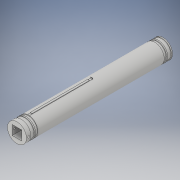
# Autodesk Inventor part: Axel_SBail
Saved by Autodesk Inventor 2019 (Build 230136000, 136)
## iProperties
Created: 2019-04-10
Part Number: Axel_SBail
Material: Generic
Document SubType Name: Modeling
Designer: samson.bailor
Density: 1 g/cm^3
Appearance: Default
Author: samson.bailor
Autodesk Inventor part; units mm, degrees
ref_plane "YZ Plane" through (0, 0, 0) normal (1, 0, 0) x (0, 1, 0)
ref_plane "XZ Plane" through (0, 0, 0) normal (0, 1, 0) x (-1, 0, 0)
ref_plane "XY Plane" through (0, 0, 0) normal (0, 0, 1) x (1, 0, 0)
sketch "Sketch1" plane through (0, 0, 0) normal (0, 0, 1) x (1, 0, 0)
  circle A0 centre (0, 0) radius 25.4
  dimension "d0" = 50.8
  constraints: 1 centre point, 1 coincident
  measures "d0" diameter of A0
extrude "Extrusion1" add sketch "Sketch1" along normal blind 355.6
sketch "Sketch4" plane through (0, 0, 355.6) normal (0, 0, 1) x (1, 0, 0)
  line L0 (31.0854, 16.4706) -> (47.788, 16.4706)
  line L1 (47.788, 16.4706) -> (47.788, 0)
  line L2 (47.788, 0) -> (31.0854, 0)
  line L3 (31.0854, 0) -> (31.0854, 16.4706)
  point P0 (0, 0)
  constraints: 8 end point, 2 parallel, 1 horizontal, 1 perpendicular
extrude "Extrusion4" add sketch "Sketch4" against normal blind 3.175
sketch "Sketch5" plane through (0, 0, 352.425) normal (0, 0, -1) x (-1, 0, 0)
  circle A0 centre (0, 0) radius 25.4
  circle A1 centre (0, 0) radius 23.8125
  dimension "d19" = 1.5875
  constraints: 2 centre point, 1 coincident
  measures "d19" radial gap between concentric circles of A0 A1
extrude "Extrusion5" cut sketch "Sketch5" along normal blind 6.35
sketch "Sketch6" plane through (0, 0, 0) normal (0, 0, -1) x (-1, 0, 0)
  line L0 (29.0417, -43.641) -> (10.5178, -43.641)
  line L1 (10.5178, -43.641) -> (10.5178, -69.3861)
  line L2 (10.5178, -69.3861) -> (29.0417, -69.3861)
  line L3 (29.0417, -69.3861) -> (29.0417, -43.641)
  point P0 (0, 0)
  constraints: 8 end point, 2 parallel, 1 horizontal, 1 perpendicular
extrude "Extrusion6" add sketch "Sketch6" against normal blind 3.175
sketch "Sketch7" plane through (0, 0, 3.175) normal (0, 0, 1) x (1, 0, 0)
  circle A0 centre (0, 0) radius 25.4
  circle A1 centre (0, 0) radius 23.8125
  constraints: 2 centre point, 2 coincident
extrude "Extrusion7" cut sketch "Sketch7" along normal blind 6.35
sketch "Sketch8" plane through (-29.0417, -69.3861, 0) normal (-1, 0, 0) x (0, 0, 1)
  line L0 (0, 0) -> (0, 25.7451) projected
  line L1 (3.175, 25.7451) -> (3.175, 0) projected
  line L2 (0, 0) -> (3.175, 0)
  line L3 (3.175, 0) -> (3.175, 25.7451)
  line L4 (3.175, 25.7451) -> (0, 25.7451)
  line L5 (0, 25.7451) -> (0, 0)
  point P0 (0, 69.3861)
  constraints: 8 end point, 2 parallel, 1 horizontal, 1 perpendicular
extrude "Extrusion8" cut sketch "Sketch8" against normal through all
sketch "Sketch9" plane through (0, 0, 355.6) normal (0, 0, 1) x (1, 0, 0)
  line L0 (31.0854, 16.4706) -> (47.788, 16.4706) projected
  line L1 (31.0854, 16.4706) -> (47.788, 16.4706)
  line L2 (47.788, 16.4706) -> (47.788, 0)
  line L3 (47.788, 0) -> (31.0854, 0)
  line L4 (31.0854, 0) -> (31.0854, 16.4706)
  point P0 (0, 0)
  constraints: 8 end point, 2 parallel, 1 horizontal, 1 perpendicular
extrude "Extrusion9" cut sketch "Sketch9" against normal blind 6.35
sketch "Sketch10" plane through (0, 0, 346.075) normal (0, 0, 1) x (1, 0, 0)
  circle A0 centre (0, 0) radius 25.4 projected
  line L0 (2.54, 25.4) -> (2.54, 26.67)
  line L1 (2.54, 26.67) -> (0, 26.67)
  line L2 (0, 26.67) -> (0, 25.4)
  line L3 (-2.54, 25.4) -> (-2.54, 26.67)
  line L4 (-2.54, 26.67) -> (0, 26.67)
  line L5 (0, 26.67) -> (0, 25.4)
  arc A1 (2.54, 25.2727) -> (-2.54, 25.2727) centre (0, 0) ccw
  line L6 (2.54, 25.4) -> (2.54, 25.2727)
  line L7 (-2.54, 25.4) -> (-2.54, 25.2727)
  dimension "d30" = 2.54
  dimension "d31" = 1.27
  dimension "d32" = 2.54
  dimension "d33" = 1.27
  constraints: 16 end point, 3 point on circle, 2 parallel, 2 vertical, 1 centre point, 1 vertical alignment, 1 other
  measures "d30" distance of L1.end L0.end
  measures "d31" distance of L0.end L0.start
  measures "d32" distance of L3.end L4.end
  measures "d33" distance of L3.start L3.end
extrude "Extrusion10" add sketch "Sketch10" against normal blind 168.275 contours A0 L2 L1 L0 L6 | L7 L3 L4 L2 A0
sketch "Sketch11" plane through (-2.54, 26.67, 346.075) normal (0, 1, 0) x (1, 0, 0)
  line L0 (5.08, 168.275) -> (0, 168.275) projected
  line L1 (0, 0) -> (0, 168.275) projected
  line L2 (5.08, 168.275) -> (0, 168.275)
  line L3 (0, 168.275) -> (0, 167.64)
  line L4 (0, 167.64) -> (5.08, 167.64)
  line L5 (5.08, 167.64) -> (5.08, 168.275)
  line L6 (5.08, 168.275) -> (0, 168.275)
  line L7 (0, 168.275) -> (0, 168.91)
  line L8 (0, 168.91) -> (5.08, 168.91)
  line L9 (5.08, 168.91) -> (5.08, 168.275)
  point P0 (2.54, 346.075)
  dimension "d36" = 0.635
  dimension "d37" = 0.635
  constraints: 16 end point, 4 parallel, 2 horizontal, 2 perpendicular, 2 point on line
  measures "d36" distance of L3.end L2.end
  measures "d37" distance of L6.end L7.end
sketch "Sketch12" plane through (0, 0, 177.8) normal (0, 0, -1) x (-1, 0, 0)
  line L0 (2.54, 26.67) -> (-2.54, 26.67) projected
  line L1 (-2.54, 26.67) -> (-2.54, 25.2727)
  line L2 (-2.54, 25.2727) -> (2.54, 25.2727)
  line L3 (2.54, 25.2727) -> (2.54, 26.67) projected
  line L4 (2.54, 26.67) -> (2.54, 25.2727)
  line L5 (-2.54, 26.67) -> (2.54, 26.67)
  arc A0 (2.54, 25.2727) -> (-2.54, 25.2727) centre (0, 0) ccw
  arc A1 (-2.54, 25.2727) -> (2.54, 25.2727) centre (0, 0) ccw projected
  arc A2 (2.54, 25.2727) -> (-2.54, 25.2727) centre (0, 0) ccw
  constraints: 8 end point, 4 point on circle, 3 perpendicular, 2 centre point, 1 vertical
extrude "Extrusion11" add sketch "Sketch12" along normal blind 0.635 contours L3 A0 L1 L0
extrude "Extrusion12" add sketch "Sketch11" along normal blind 1.27
sketch "Sketch13" plane through (0, 0, 355.6) normal (0, 0, 1) x (1, 0, 0)
  line L0 (13.9466, 0.955) -> (12.6912, 0.4731) projected
  line L1 (13.8404, 1.9655) -> (13.9466, 0.955) projected
  circle A0 centre (0, 0) radius 13.9792
  circle A1 centre (0, 0) radius 25.4
  circle A2 centre (0, 0) radius 23.8125 projected
  circle A3 centre (0, 0) radius 23.8125
  constraints: 2 centre point, 2 coincident, 3 other
extrude "Extrusion13" add sketch "Sketch13" along normal blind 9.525 contours A2
sketch "Sketch14" plane through (0, 0, 365.125) normal (0, 0, 1) x (1, 0, 0)
  circle A0 centre (0, 0) radius 25.4
  arc A1 (13.9792, 0) -> (13.9792, 0) centre (0, 0) ccw projected
  circle A2 centre (0, 0) radius 13.9792
  constraints: 2 coincident, 1 centre point, 1 horizontal alignment, 2 other
extrude "Extrusion14" add sketch "Sketch14" along normal blind 3.175
sketch "Sketch16" plane through (0, 0, 0) normal (0, 0, -1) x (-1, 0, 0)
  circle A0 centre (0, 0) radius 23.8125
  circle A1 centre (0, 0) radius 13.9792
  point P0 (-13.9792, 0)
  point P1 (-13.9792, 0)
  constraints: 2 coincident, 1 centre point, 1 horizontal alignment, 2 other
extrude "Extrusion15" add sketch "Sketch16" along normal blind 9.525
sketch "Sketch17" plane through (0, 0, -9.525) normal (0, 0, -1) x (-1, 0, 0)
  circle A0 centre (0, 0) radius 25.4
  line L0 (8.8437, -9.1148) -> (9.2337, -9.3135) projected
  circle A1 centre (0, 0) radius 13.9792
  point P0 (13.9792, 0)
  constraints: 2 coincident, 1 centre point, 1 horizontal alignment, 2 other
extrude "Extrusion16" add sketch "Sketch17" along normal blind 3.175
sketch "Sketch18" plane through (-2.54, 26.67, 346.075) normal (0, 1, 0) x (1, 0, 0)
  line L0 (5.08, 168.91) -> (5.08, 0) projected
  line L1 (0, 0) -> (5.08, 0)
  line L2 (5.08, 0) -> (5.08, 7.62)
  line L3 (5.08, 7.62) -> (0, 7.62)
  line L4 (0, 7.62) -> (0, 0)
  line L5 (0, 167.64) -> (5.08, 167.64) projected
  line L6 (0, 0) -> (0, 168.91) projected
  line L7 (5.08, 167.64) -> (0, 167.64)
  line L8 (0, 167.64) -> (0, 160.02)
  line L9 (0, 160.02) -> (5.08, 160.02)
  line L10 (5.08, 160.02) -> (5.08, 167.64)
  point P0 (2.54, 346.075)
  dimension "d50" = 7.62
  dimension "d51" = 7.62
  constraints: 16 end point, 4 parallel, 2 horizontal, 2 perpendicular, 2 point on line
  measures "d50" distance of L2.end L1.end
  measures "d51" distance of L8.end L7.end
extrude "Extrusion17" cut sketch "Sketch18" against normal blind 1.27 contours L0 L9 L6 L5 | L0 L1 L4 L3
sketch "Sketch19" plane through (0, 0, 368.3) normal (0, 0, 1) x (1, 0, 0)
  circle A0 centre (0, 0) radius 15.0616
  constraints: 1 centre point, 1 coincident
extrude "Extrusion18" add sketch "Sketch19" against normal blind 25.4
sketch "Sketch20" plane through (0, 0, 368.3) normal (0, 0, 1) x (1, 0, 0)
  line L0 (0, 0) -> (-25.4, 0)
  circle A0 centre (0, 0) radius 25.4 projected
  arc A1 (-12.6912, 0.4731) -> (-12.6912, -0.4731) centre (0, 0) ccw projected
  line L1 (-12.7, 0) -> (-12.7, 12.7)
  line L2 (-12.7, 12.7) -> (12.7, 12.7)
  line L3 (12.7, 12.7) -> (12.7, -12.7)
  line L4 (12.7, -12.7) -> (-12.7, -12.7)
  line L5 (-12.7, -12.7) -> (-12.7, 0)
  dimension "d56" = 12.7
  dimension "d57" = 25.4
  dimension "d58" = 25.4
  dimension "d59" = 25.4
  constraints: 12 end point, 4 perpendicular, 2 tangent, 1 horizontal, 1 horizontal alignment, 1 midpoint, 1 point on circle, 1 point on line, 1 other
  measures "d56" distance of L1.start L1.end
  measures "d57" distance of L1.end L2.end
  measures "d58" distance of L2.end L3.end
  measures "d59" distance of L3.end L4.end
extrude "Extrusion19" cut sketch "Sketch20" against normal blind 50.8 contours L1 L2 L3 L4 L5
sketch "Sketch24" plane through (0, 0, 368.3) normal (0, 0, 1) x (1, 0, 0)
  circle A0 centre (0, 0) radius 25.4
  line L0 (12.7, 12.7) -> (12.7, -12.7) projected
  line L1 (-12.7, -12.7) -> (-12.7, 12.7) projected
  line L2 (12.7, -12.7) -> (-12.7, -12.7)
  line L3 (-12.7, -12.7) -> (-12.7, 12.7)
  line L4 (-12.7, 12.7) -> (12.7, 12.7)
  line L5 (12.7, 12.7) -> (12.7, -12.7)
  constraints: 8 end point, 2 parallel, 1 centre point, 1 coincident, 1 horizontal, 1 perpendicular
extrude "Extrusion24" add sketch "Sketch24" along normal blind 8.382
sketch "Sketch25" plane through (-12.7, -12.7, 317.5) normal (1, 0, 0) x (0, 0, -1)
  line L0 (-47.625, 38.1) -> (-59.182, 38.1) projected
  line L1 (-53.4035, 38.1) -> (-53.4035, -12.7)
  line L2 (-47.625, -12.7) -> (-59.182, -12.7) projected
  circle A0 centre (-53.4035, 12.7) radius 2.54
  point P0 (317.5, 12.7)
  dimension "d73" = 5.08
  constraints: 3 midpoint, 2 end point, 1 centre point
  measures "d73" diameter of A0
extrude "Extrusion25" cut sketch "Sketch25" against normal blind 8.382
extrude "Extrusion26" cut sketch "Sketch25" along normal blind 50.8
body "Solid1"
